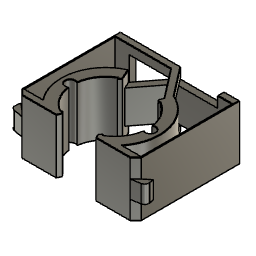
omega clamp (Autodesk Fusion 360 design; units mm, degrees)
Autodesk Fusion 360 part; units mm, degrees
sketch "Sketch1" plane through (0, 0, 0) normal (0, 0, 1) x (1, 0, 0)
  circle A0 centre (0, 0) radius 14.3
  line L0 (-7.1153, 12.4042) -> (-7.4636, 13.0113)
  arc A1 (-7.4636, 13.0113) -> (-14.8873, 1.8356) centre (0, 0) ccw
  arc A2 (-14.8873, 1.8356) -> (-14.8873, -1.8356) centre (-16.1, 0) ccw
  arc A3 (-14.8873, -1.8356) -> (-7.4636, -13.0113) centre (0, 0) ccw
  line L1 (-7.4636, -13.0113) -> (-7.1153, -12.4042)
  line L2 (0, 0) -> (-44, 0) construction
  line L3 (-7.1153, -12.4042) -> (-7.1153, 12.4042) construction
  line L4 (-5.7768, -13.0812) -> (-8.2006, -18.5699)
  line L5 (-5.7768, 13.0812) -> (-8.2006, 18.5699)
  arc A4 (-8.2006, 18.5699) -> (-8.2006, -18.5699) centre (0, 0) ccw
  line L6 (-7.1153, 12.4042) -> (-6.0192, 13.6301)
  line L7 (-7.1153, -12.4042) -> (-6.0192, -13.6301)
  point P0 (-18.3, 0)
  point P1 (-14.3, 0)
  point P2 (-20.3, 0)
  dimension "d8" = 0.7
  dimension "d12" = 2.2
  dimension "d13" = 120.321
  dimension "d14" = 4
  dimension "d15" = 2
  dimension "d16" = 1.5
  dimension "d76" = 0.6
  dimension "d77" = 0.6
  dimension "d80" = 30
  constraint coincident A0.centre A1.centre
  constraint coincident A0 L0.start
  constraint coincident A0.centre L0
  constraint coincident A0 L1.end
  constraint coincident A0.centre L1
  constraint horizontal L2
  constraint coincident A2.centre L2
  constraint equal L0 L1
  constraint midpoint A2 P0
  constraint coincident A0 P1
  constraint coincident L2 P1
  constraint vertical L3
  constraint coincident A0 L4.start
  constraint coincident A0.centre L4
  constraint coincident A0 L5.start
  constraint coincident L5 A0.centre
  constraint coincident L2 P2
  constraint coincident A4 P2
  constraint midpoint A4 P2
  constraint coincident L5 L6.end
  constraint coincident L4 L7.end
  measures "d8" distance of L0.start L0.end
  measures "d12" radius of A2
  measures "d13" angle of L0 L1
  measures "d14" distance of P0 P1
  measures "d15" distance of P0 P2
  measures "d16" distance of L0.start L5.start
  measures "d76" distance of L5.start L6.end
  measures "d77" distance of L4.start L7.end
  measures "d80" diameter of A1
extrude "Extrude1" add sketch "Sketch1" along normal blind 25 contours L0 A1 A2 A3 L1 L4 L5 A4 L6 L7 makes body 1
ref_plane "WorkPlane1" through (-14.8873, 1.8356, 12.5) normal (-1, 0, 0) x (0, 0, 1)
ref_plane "WorkPlane2" through (2.1127, 1.8356, 12.5) normal (-1, 0, 0) x (0, 0, 1)
mirror "Mirror1" about plane through (2.1127, 1.8356, 12.5) normal (-1, 0, 0) of bodies 1 makes body 2
sketch "Sketch2" plane through (0, 0, 0) normal (0, 0, 1) x (1, 0, 0)
  line L0 (-6.0192, 13.6301) -> (-8.2006, 18.5699)
  arc A0 (-8.2006, 18.5699) -> (-8.2006, -18.5699) centre (0, 0) ccw
  line L1 (-8.2006, -18.5699) -> (-6.0192, -13.6301)
  line L2 (-7.1153, -12.4042) -> (-7.4636, -13.0113)
  arc A1 (-14.8873, -1.8356) -> (-7.4636, -13.0113) centre (0, 0) ccw
  arc A2 (-14.8873, 1.8356) -> (-14.8873, -1.8356) centre (-16.1, 0) ccw
  arc A3 (-7.4636, 13.0113) -> (-14.8873, 1.8356) centre (0, 0) ccw
  line L3 (-7.4636, 13.0113) -> (-7.1153, 12.4042)
  line L4 (12.4261, 18.5699) -> (10.2446, 13.6301)
  line L5 (11.3407, 12.4042) -> (11.689, 13.0113)
  arc A4 (19.1127, 1.8356) -> (11.689, 13.0113) centre (4.2255, 0) ccw
  arc A5 (19.1127, -1.8356) -> (19.1127, 1.8356) centre (20.3255, 0) ccw
  arc A6 (11.689, -13.0113) -> (19.1127, -1.8356) centre (4.2255, 0) ccw
  line L6 (11.689, -13.0113) -> (11.3407, -12.4042)
  line L7 (10.2446, -13.6301) -> (12.4261, -18.5699)
  arc A7 (12.4261, -18.5699) -> (12.4261, 18.5699) centre (4.2255, 0) ccw
  line L8 (-13.0257, -15.5699) -> (-24.9401, -15.5699)
  line L9 (-24.9401, -15.5699) -> (-24.9401, -12.5699)
  line L10 (-24.9401, -12.5699) -> (-15.9401, -12.5699)
  line L11 (-24.9401, -12.5699) -> (-24.9401, 28.5699)
  line L12 (-24.3401, 28.5699) -> (-24.3401, -12.5699)
  line L13 (-24.9401, 28.5699) -> (0.9489, 28.5699)
  line L14 (-24.9401, 28.5699) -> (-24.9401, 31.5699)
  line L15 (-24.9401, 31.5699) -> (2.4261, 31.5699)
  line L16 (2.4261, 31.5699) -> (12.4261, 18.5699)
  line L17 (0.9489, 28.5699) -> (11.0457, 15.444)
  line L18 (-13.0257, -15.5699) -> (-6.8758, -15.5699)
  line L19 (-22.4401, -15.5699) -> (-24.9401, -13.0699)
  line L20 (-6.8758, -15.5699) -> (36, -15.5699)
  line L21 (-7.1153, 12.4042) -> (-6.0192, 13.6301)
  line L22 (-6.0192, -13.6301) -> (-7.1153, -12.4042)
  line L23 (10.2446, 13.6301) -> (11.3407, 12.4042)
  line L24 (11.3407, -12.4042) -> (10.2446, -13.6301)
  dimension "d40" = 3
  dimension "d41" = 0.6
  dimension "d42" = 3
  dimension "d43" = 3
  dimension "d45" = 10
  dimension "d46" = 10
  dimension "d47" = 41.1397
  dimension "d48" = 9
  dimension "d49" = 45
  dimension "d50" = 0.5
  dimension "d51" = 3
  constraint coincident A0 L8.start
  constraint horizontal L8
  constraint perpendicular L8 L9
  constraint coincident A0 L10.end
  constraint perpendicular L9 L10
  constraint perpendicular L10 L11
  constraint coincident L10 L12.end
  constraint perpendicular L10 L12
  constraint perpendicular L12 L13
  constraint coincident L12.start L13
  constraint perpendicular L13 L14
  constraint perpendicular L14 L15
  constraint coincident L4.start A7.end
  constraint coincident L4 L17.end
  constraint parallel L16 L17
  constraint coincident L1 L18.end
  constraint horizontal L18
  constraint coincident L8 L19.start
  constraint coincident L9 L19.end
  constraint parallel L18 L20
  measures "d40" distance of L8.end L9.end
  measures "d41" distance of L11 L12
  measures "d42" distance of L16 L17
  measures "d43" distance of L13 L15
  measures "d45" horizontal distance of L15.end L4.start
  measures "d46" vertical distance of L0.end L13.end
  measures "d47" distance of L9.end L11.end
  measures "d48" distance of L9.end L10.end
  measures "d49" angle of L8 L19
  measures "d50" distance of L9.end L19.end
  measures "d51" vertical distance of A0.end L8.start
extrude "Extrude2" add sketch "Sketch2" along normal up to surface (25 mm away) separate body contours A0 L8 L9 L10 L19 | L10 L11 L12 L13 | L4 L13 L14 L15 L16 L17 makes body 3
extrude "Extrude4" cut sketch "Sketch2" along normal up to surface (25 mm away) contours A0 L1 L18 | L7 A7 L20 bodies 1 2
ref_plane "WorkPlane3" through (-6.257, 8, 12.5) normal (0, 0, 1) x (1, 0, 0)
sketch "Sketch4" plane through (-6.4898, 5.5, 12.5) normal (0, 0, 1) x (1, 0, 0)
  line L0 (-17.8503, -18.0699) -> (-17.8503, 23.0699)
  line L1 (-17.8503, 23.0699) -> (7.4387, 23.0699)
  line L2 (7.4387, 23.0699) -> (17.5355, 9.944)
  line L3 (17.5355, 9.944) -> (18.9159, 13.0699)
  line L4 (18.9159, 13.0699) -> (8.9159, 26.0699)
  line L5 (8.9159, 26.0699) -> (-18.4503, 26.0699)
  line L6 (-18.4503, 26.0699) -> (-18.4503, -18.5699)
  line L7 (-18.4503, -18.5699) -> (-15.9503, -21.0699)
  line L8 (-15.9503, -21.0699) -> (-6.5359, -21.0699)
  arc A0 (-9.4503, -18.0699) -> (-6.5359, -21.0699) centre (6.4898, -5.5) ccw
  line L9 (-9.4503, -18.0699) -> (-17.8503, -18.0699)
  line L10 (-15.9503, -21.0699) -> (-20.1729, -20.3253)
  line L11 (-21.7952, -18.0084) -> (-21.4503, -16.0526)
  line L12 (-21.4503, -16.0526) -> (-18.4503, -18.5699)
  arc A1 (-21.7952, -18.0084) -> (-20.1729, -20.3253) centre (-19.8256, -18.3557) ccw
  dimension "d69" = 2
  dimension "d70" = 3
  dimension "d72" = 50
  dimension "d73" = 10
  constraint coincident L7.end L8.start
  constraint perpendicular L10 L11
  constraint coincident L6.end L7.start
  constraint tangent L10 A1
  constraint tangent L11 A1
  measures "d69" radius of A1
  measures "d70" horizontal distance of L11.end L6.end
  measures "d72" angle of L6 L12
  measures "d73" angle of L8 L10
extrude "Extrude7" add sketch "Sketch4" along normal mid plane 8 contours L7 L10 L11 L12 A1 bodies 3
mirror "Mirror2" about plane through (2.1127, 1.8356, 12.5) normal (-1, 0, 0) of bodies 3 makes body 4
sketch "Sketch3" plane through (0, 31.5699, 0) normal (0, 1, 0) x (-1, 0, 0)
  line L0 (-1.7994, 25) -> (-29.1656, 25)
  line L1 (-29.1656, 0) -> (-1.7994, 0)
  line L2 (24.9401, 25) -> (-2.4261, 25)
  line L3 (-2.4261, 0) -> (24.9401, 0)
  line L4 (24.9401, 4) -> (-29.1656, 4)
  line L5 (24.9401, 5) -> (-29.1656, 5)
  line L6 (-29.1656, 20) -> (24.9401, 20)
  line L7 (24.9401, 21) -> (-29.1656, 21)
  line L8 (-2.1127, 4) -> (-2.1127, 5) construction
  line L9 (-2.1127, 20) -> (-2.1127, 21) construction
  line L10 (-2.1127, 21) -> (-2.1127, 25) construction
  line L11 (-2.1127, 4) -> (-2.1127, 0) construction
  line L12 (8.2006, 25) -> (-1.7994, 25)
  line L13 (-1.7994, 0) -> (8.2006, 0)
  line L14 (-29.1656, 25) -> (-29.1656, 0)
  line L15 (24.9401, 0) -> (24.9401, 25)
  line L16 (17.8873, 25) -> (17.8873, 0)
  line L17 (-22.1127, 0) -> (-22.1127, 25)
  line L18 (-22.1127, 0) -> (17.8873, 0) construction
  dimension "d58" = 1
  dimension "d59" = 4
  dimension "d78" = 40
  constraint midpoint L4 L8.start
  constraint midpoint L5 L8.end
  constraint midpoint L6 L9.start
  constraint midpoint L7 L9.end
  constraint perpendicular L7 L10
  constraint perpendicular L4 L11
  constraint equal L10 L11
  constraint equal L8 L9
  constraint coincident L11.end L13
  constraint coincident L10.end L12
  constraint coincident L7.start L15
  constraint perpendicular L7 L15
  constraint coincident L6.end L15
  constraint coincident L7.end L14
  constraint coincident L6.start L14
  constraint horizontal L6
  constraint coincident L5.start L15
  constraint perpendicular L5 L15
  constraint vertical L8
  constraint coincident L4.end L14
  constraint coincident L5.end L14
  constraint coincident L2 L16.start
  constraint coincident L3 L16.end
  constraint perpendicular L3 L16
  constraint coincident L1 L17.start
  constraint coincident L0 L17.end
  constraint perpendicular L0 L17
  constraint coincident L17 L18.start
  constraint coincident L16 L18.end
  constraint perpendicular L16 L18
  constraint midpoint L11.end L18
  measures "d58" distance of L4 L5
  measures "d59" distance of L9.end L10.end
  measures "d78" distance of L17.start L16.end
extrude "Extrude5" cut sketch "Sketch3" against normal blind 20 contours L0 L2 L7 L12 L16 L17 | L6 L7 L16 L17 | L4 L5 L16 L17 | L1 L3 L4 L13 L16 L17 bodies 4
extrude "Extrude6" cut sketch "Sketch3" against normal blind 25 contours L6 L7 L16 L17 | L5 L6 L16 L17 | L4 L5 L16 L17 bodies 3
combine "Combine1" operation add target body 1 tool bodies 2 3 4
chamfer "Chamfer3" distance 0.2 angle 45 2 faces at (19.3108, -14.5699, 0) (19.3108, -14.5699, 25) on bodies 1
equation "rubber_width = 29.5 mm"
equation "shaft_diameter = 30 mm"
equation "chord_angle = ( ( rubber_width + slop ) / ( shaft_diameter * PI ) * 2 * PI ) * 1 rad"
equation "d13 = chord_angle"
equation "d80 = shaft_diameter"
equation "slop = 2 mm"
